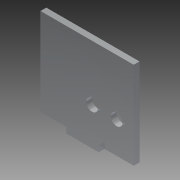
# Autodesk Inventor part: Side B
Saved by Autodesk Inventor 2014 (Build 180170000, 170)
## iProperties
Created: 2014-11-21
Part Number: Side B
Material: Generic
Document SubType Name: Modeling
Designer: JLM
Density: 1 g/cm^3
Appearance: Default
Author: JLM
Autodesk Inventor part; units mm, degrees
ref_plane "YZ Plane" through (0, 0, 0) normal (1, 0, 0) x (0, 1, 0)
ref_plane "XZ Plane" through (0, 0, 0) normal (0, 1, 0) x (-1, 0, 0)
ref_plane "XY Plane" through (0, 0, 0) normal (0, 0, 1) x (1, 0, 0)
sketch "Sketch1" plane through (0, 0, 0) normal (0, 0, 1) x (1, 0, 0)
  line L0 (-25.4, -25.4) -> (25.4, -25.4)
  line L1 (25.4, -25.4) -> (25.4, 25.4)
  line L2 (25.4, 25.4) -> (-25.4, 25.4)
  line L3 (-25.4, 25.4) -> (-25.4, -25.4)
  line L4 (-25.4, -25.4) -> (25.4, 25.4) construction
  line L5 (25.4, -25.4) -> (-25.4, 25.4) construction
  point P0 (0, 0)
  dimension "d0" = 50.8
  dimension "d1" = 50.8
  constraints: 12 end point, 2 midpoint, 2 parallel, 1 horizontal, 1 perpendicular
  measures "d0" distance of L2.end L1.end
  measures "d1" distance of L1.end L0.end
extrude "Extrusion1" add sketch "Sketch1" against normal blind 3.175
sketch "Sketch4" plane through (0, 0, 0) normal (0, 0, 1) x (1, 0, 0)
  line L0 (25.4, -22.2383) -> (9.525, -22.2383)
  line L1 (9.525, -22.2383) -> (9.525, -25.4133)
  line L2 (9.525, -25.4133) -> (25.4, -25.4133)
  line L3 (25.4, -25.4133) -> (25.4, -22.2383)
  line L4 (-25.4, -25.4) -> (-9.525, -25.4)
  line L5 (-9.525, -25.4) -> (-9.525, -22.225)
  line L6 (-9.525, -22.225) -> (-25.4, -22.225)
  line L7 (-25.4, -22.225) -> (-25.4, -25.4)
  line L8 (25.4, -25.4) -> (25.4, 25.4) projected
  line L9 (25.4, 25.4) -> (-25.4, 25.4) projected
  line L10 (-25.4, 25.4) -> (-25.4, -25.4) projected
  line L11 (-25.4, 19.05) -> (-22.225, 19.05)
  line L12 (-22.225, 19.05) -> (-22.225, 0)
  line L13 (-22.225, 0) -> (-25.4, 0)
  line L14 (-25.4, 0) -> (-25.4, 19.05)
  line L15 (25.4, 19.05) -> (22.225, 19.05)
  line L16 (22.225, 19.05) -> (22.225, 0)
  line L17 (22.225, 0) -> (25.4, 0)
  line L18 (25.4, 0) -> (25.4, 19.05)
  line L19 (-9.525, 25.4) -> (9.525, 25.4)
  line L20 (9.525, 25.4) -> (9.525, 22.225)
  line L21 (9.525, 22.225) -> (-9.525, 22.225)
  line L22 (-9.525, 22.225) -> (-9.525, 25.4)
  point P0 (0, 0)
  dimension "d12" = 15.875
  dimension "d13" = 3.175
  dimension "d16" = 3.175
  dimension "d37" = 9.525
  dimension "d38" = 15.875
  dimension "d39" = 9.525
  dimension "d40" = 3.175
  dimension "d41" = 3.175
  dimension "d42" = 19.05
  dimension "d43" = 19.05
  dimension "d44" = 3.175
  dimension "d45" = 19.05
  dimension "d46" = 15.875
  constraints: 40 end point, 10 parallel, 5 horizontal, 5 perpendicular, 3 point on line
  measures "d12" distance of L2.end L1.end
  measures "d13" distance of L1.end L0.end
  measures "d16" distance of L4.end L5.end
  measures "d37" distance from line of point (0, 0) L5
  measures "d38" distance of L4.start L4.end
  measures "d39" distance from line of point (0, 0) L1
  measures "d40" distance of L11.start L11.end
  measures "d41" distance of L15.start L15.end
  measures "d42" distance of L11.end L12.end
  measures "d43" distance of L15.end L16.end
  measures "d44" distance of L21.end L19.start
  measures "d45" distance of L20.end L21.end
  measures "d46" distance between parallel lines of L10 L22
extrude "Extrusion5" cut sketch "Sketch4" against normal blind 25.4
hole "Hole1" at (0, 0, 0) direction (0, 0, -1) diameter 19.05 end through all
hole "Hole2" at (15.653, -11.4451, 0) direction (0, 0, -1) diameter 6.35 end through all
equation "\"d12\" = d38"
equation "\"d13\" = d16"
equation "\"d38\" = -d37 + 0.5 * d0"
equation "\"d39\" = d37"
equation "\"d40\" = d16"
equation "\"d41\" = d16"
equation "\"d42\" = 2 * d37"
equation "\"d43\" = d42"
equation "\"d44\" = d16"
equation "\"d45\" = d42"
equation "\"d46\" = d38"
equation "\"d48\" = 0.5 * d0"
body "Solid1"
